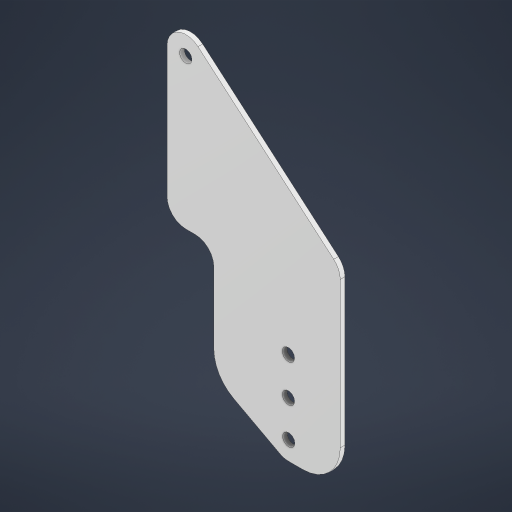
# Autodesk Inventor part: back_sled
Saved by Autodesk Inventor 2024 (Build 280153000, 153)
## iProperties
Created: 2024-01-16
Part Number: back_sled
Material: Acetal Resin, White
Document SubType Name: Modeling
Designer: avere
Density: 1.425 g/cm^3
Appearance: Smooth - White
Author: avere
Autodesk Inventor part; units mm, degrees
ref_plane "YZ Plane" through (0, 0, 0) normal (1, 0, 0) x (0, 1, 0)
ref_plane "XZ Plane" through (0, 0, 0) normal (0, 1, 0) x (-1, 0, 0)
ref_plane "XY Plane" through (0, 0, 0) normal (0, 0, 1) x (1, 0, 0)
sketch "main" plane through (0, 0, 0) normal (0, 0, 1) x (1, 0, 0)
  arc A0 (-13.083, -30.8821) -> (-6.3594, -42.088) centre (-0.383, -30.8821) ccw
  line L0 (-13.083, -6.7521) -> (-13.083, -30.8821)
  arc A1 (-13.083, -6.7521) -> (-19.433, -0.4021) centre (-19.433, -6.7521) ccw
  line L1 (-6.3594, -42.088) -> (9.3288, -50.4551)
  line L2 (29.7795, 10.9635) -> (29.7795, -38.5021)
  arc A2 (29.7795, 10.9635) -> (27.5605, 15.7861) centre (23.4295, 10.9635) ccw
  circle A3 centre (12.317, -44.8521) radius 2.0955
  arc A4 (9.3288, -50.4551) -> (12.317, -51.2021) centre (12.2103, -45.2792) ccw
  line L3 (17.0795, -51.2021) -> (12.317, -51.2021)
  arc A5 (17.0795, -51.2021) -> (29.7795, -38.5021) centre (17.0795, -38.5021) ccw
  circle A6 centre (-22.608, 50.3979) radius 2.0955
  arc A7 (-18.477, 55.2205) -> (-28.958, 50.3979) centre (-22.608, 50.3979) ccw
  line L4 (27.5605, 15.7861) -> (-18.477, 55.2205)
  line L5 (-22.608, -0.4021) -> (-19.433, -0.4021)
  arc A8 (-28.958, 5.9479) -> (-22.608, -0.4021) centre (-22.608, 5.9479) ccw
  line L6 (-28.958, 50.3979) -> (-28.958, 5.9479)
  point P0 (-1.5201, -8.3134)
  dimension "d1" = 4.191
  dimension "d2" = 12.7
  dimension "d3" = 4.191
  dimension "d4" = 12.7
  dimension "d5" = 12.7
  dimension "d6" = 6.35
  dimension "d7" = 6.35
  measures "d1" diameter of A6
  measures "d2" diameter of A7
  measures "d3" diameter of A3
  measures "d4" radius of A5
  measures "d5" radius of A0
  measures "d6" radius of A1
  measures "d7" radius of A2
sketch "Sketch1" plane through (0, 0, 0) normal (0, 0, 1) x (1, 0, 0)
  circle A0 centre (-0.1068, 24.9729) radius 2.0955
  circle A1 centre (-0.1068, 12.2729) radius 2.0955
  arc A2 (-25.4, 13.97) -> (-18.6765, 2.7641) centre (-12.7, 13.97) ccw
  line L0 (-25.4, 38.1) -> (-25.4, 13.97)
  arc A3 (-25.4, 38.1) -> (-31.75, 44.45) centre (-31.75, 38.1) ccw
  line L1 (-18.6765, 2.7641) -> (-2.9882, -5.6029)
  line L2 (17.4625, 55.8156) -> (17.4625, 6.35)
  arc A4 (17.4625, 55.8156) -> (15.2434, 60.6383) centre (11.1125, 55.8156) ccw
  circle A5 centre (0, 0) radius 2.0955
  arc A6 (-2.9882, -5.6029) -> (0, -6.35) centre (-0.1068, -0.4271) ccw
  line L3 (4.7625, -6.35) -> (0, -6.35)
  arc A7 (4.7625, -6.35) -> (17.4625, 6.35) centre (4.7625, 6.35) ccw
  circle A8 centre (-34.925, 95.25) radius 2.0955
  arc A9 (-30.7941, 100.0726) -> (-41.275, 95.25) centre (-34.925, 95.25) ccw
  line L4 (15.2434, 60.6383) -> (-30.7941, 100.0726)
  line L5 (-34.925, 44.45) -> (-31.75, 44.45)
  arc A10 (-41.275, 50.8) -> (-34.925, 44.45) centre (-34.925, 50.8) ccw
  line L6 (-41.275, 95.25) -> (-41.275, 50.8)
  dimension "d11" = 4.191
  dimension "d12" = 4.191
  constraints: 2 centre point, 1 other
  measures "d11" diameter of A0
  measures "d12" diameter of A1
extrude "Extrusion1" add sketch "Sketch1" along normal blind 1.5875
body "Solid1"
